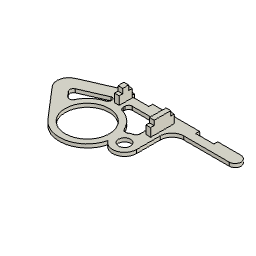
Prototype Body improved v2 (Autodesk Fusion 360 archive; units mm, degrees)
design "bottom_chassis"
Autodesk Fusion 360 part; units mm, degrees
(part 1 of 6)
sketch "Sketch1" plane through (0, 0, 0) normal (0, 0, 1) x (1, 0, 0)
  circle A0 centre (0, 0) radius 18.6
  line L0 (-40.1145, 10.4906) -> (-17.9049, -15.3744)
  line L1 (5, 25.3685) -> (5, 26.9321)
  line L2 (-5, 26.019) -> (-5, 25.3685)
  line L3 (-5, 40) -> (-36.5447, 26.1628)
  line L4 (-28.8171, 18.6328) -> (-7.8034, 27.8505)
  line L5 (-29.888, 13.9311) -> (-26.2116, 9.6495)
  arc A1 (-36.5447, 26.1628) -> (-40.1145, 10.4906) centre (-32.5276, 17.0051) ccw
  line L6 (15.2, 40) -> (15.2, 36.8)
  line L7 (15.2, 36.8) -> (0, 36.8)
  line L8 (0, 36.8) -> (0, 40)
  line L9 (15.2, 40) -> (55, 40)
  line L10 (70.2, 40) -> (70.2, 36.8)
  line L11 (70.2, 36.8) -> (55, 36.8)
  line L12 (55, 36.8) -> (55, 40)
  line L13 (-5, 40) -> (0, 40)
  line L14 (41.6, 0) -> (41.6, 20)
  arc A2 (90, 30) -> (90, 40) centre (90, 35) ccw
  line L15 (90, 30) -> (51.6, 30)
  line L16 (8, 29.9321) -> (28.6, 29.9321)
  line L17 (31.6, 26.9321) -> (31.6, 12.775)
  arc A3 (-17.9049, -15.3744) -> (22.9714, -5.4105) centre (0, 0) ccw
  arc A4 (21.5214, 9.6845) -> (7.0977, 22.5074) centre (0, 0) ccw
  arc A5 (-7.0977, 22.5074) -> (-21.236, 10.2952) centre (0, 0) ccw
  arc A6 (22.9714, -5.4105) -> (41.6, 0) centre (31.5, 0) ccw
  arc A7 (29.2641, 9.8494) -> (25.9158, 8.4159) centre (31.5, 0) ccw
  arc A8 (-28.8171, 18.6328) -> (-29.888, 13.9311) centre (-27.612, 15.8855) ccw
  arc A9 (-26.2116, 9.6495) -> (-21.236, 10.2952) centre (-23.9355, 11.6039) ccw
  arc A10 (-7.0977, 22.5074) -> (-5, 25.3685) centre (-8, 25.3685) ccw
  arc A11 (-5, 26.019) -> (-7.8034, 27.8505) centre (-7, 26.019) ccw
  arc A12 (8, 29.9321) -> (5, 26.9321) centre (8, 26.9321) ccw
  arc A13 (5, 25.3685) -> (7.0977, 22.5074) centre (8, 25.3685) ccw
  arc A14 (21.5214, 9.6845) -> (25.9158, 8.4159) centre (24.2571, 10.9156) ccw
  arc A15 (29.2641, 9.8494) -> (31.6, 12.775) centre (28.6, 12.775) ccw
  arc A16 (31.6, 26.9321) -> (28.6, 29.9321) centre (28.6, 26.9321) ccw
  arc A17 (51.6, 30) -> (41.6, 20) centre (51.6, 20) ccw
  line L18 (0, 40) -> (-5, 40)
  line L19 (90, 40) -> (70.2, 40)
  line L20 (55, 40) -> (15.2, 40)
  line L21 (-2, 36) -> (2, 36)
  line L22 (2, 36) -> (2, 25)
  line L23 (2, 25) -> (-2, 25)
  line L24 (-2, 25) -> (-2, 36)
  line L25 (-2, 33) -> (2, 33)
  line L26 (2, 33) -> (2, 28)
  line L27 (2, 28) -> (-2, 28)
  line L28 (-2, 28) -> (-2, 33)
  line L29 (34.6, 35) -> (38.6, 35)
  line L30 (38.6, 35) -> (38.6, 15)
  line L31 (38.6, 15) -> (34.6, 15)
  line L32 (34.6, 15) -> (34.6, 35)
  line L33 (34.6, 32) -> (38.6, 32)
  line L34 (34.6, 18) -> (38.6, 18)
  circle A18 centre (31.5, 0) radius 5.1
  dimension "d4" = 37.2
  dimension "d6" = 47.2
  dimension "d7" = 20.2
  dimension "d8" = 20
  dimension "d11" = 31.5
  dimension "d12" = 15.2
  dimension "d13" = 3.2
  dimension "d14" = 55
  dimension "d15" = 15.2
  dimension "d16" = 3.2
  dimension "d19" = 3
  dimension "d20" = 2
  dimension "d21" = 3
  dimension "d22" = 10
  dimension "d26" = 4
  dimension "d27" = 20
  dimension "d35" = 10.2
  constraint coincident A0.centre A3.centre
  constraint coincident L0.end A4
  constraint tangent L0 A4
  constraint tangent L0 A1
  constraint parallel L0 L5
  constraint tangent L3 A1
  constraint vertical L6
  constraint horizontal L7
  constraint vertical L8
  constraint perpendicular L6 L9
  constraint vertical L10
  constraint horizontal L11
  constraint vertical L12
  constraint tangent L14 A6
  constraint perpendicular L9 L14
  constraint tangent A2 L19
  constraint tangent A2 L15
  constraint perpendicular L14 L15
  constraint concentric A3 A4
  constraint concentric A4 A5
  constraint concentric A6 A7
  constraint tangent L4 A8
  constraint tangent L5 A8
  constraint tangent L5 A9
  constraint tangent A5 A9
  constraint equal A8 A9
  constraint tangent L2 A10
  constraint tangent A5 A10
  constraint equal A8 A10
  constraint tangent L4 A11
  constraint tangent L2 A11
  constraint tangent L16 A12
  constraint tangent L1 A12
  constraint tangent L1 A13
  constraint tangent A4 A13
  constraint equal A12 A13
  constraint tangent A4 A14
  constraint tangent A7 A14
  constraint equal A12 A14
  constraint tangent L17 A15
  constraint tangent A7 A15
  constraint equal A12 A15
  constraint tangent L16 A16
  constraint tangent L17 A16
  constraint equal A12 A16
  constraint tangent L15 A17
  constraint tangent L14 A17
  constraint collinear L18 L19
  constraint collinear L19 L20
  constraint horizontal L21
  constraint vertical L22
  constraint horizontal L23
  constraint vertical L24
  constraint horizontal L25
  constraint vertical L26
  constraint horizontal L27
  constraint vertical L28
  constraint coincident L22 L26.end
  constraint coincident L24 L25.start
  constraint horizontal L29
  constraint vertical L30
  constraint horizontal L31
  constraint vertical L32
  constraint perpendicular L32 L33
  constraint perpendicular L32 L34
  constraint coincident L30 L34.end
  constraint coincident L32 L34.start
  constraint coincident L32 L33.start
  constraint coincident L30 L33.end
  constraint concentric A6 A18
  measures "d4" diameter of A0
  measures "d6" diameter of A4
  measures "d7" diameter of A6
  measures "d8" diameter of A1
  measures "d11" distance of A0.centre A6.centre
  measures "d12" distance of L8.end L6.start
  measures "d13" distance of L8.end L7.end
  measures "d14" distance of L8.end L9.end
  measures "d15" distance of L9.end L10.start
  measures "d16" distance of L9.end L11.end
  measures "d19" radius of A8
  measures "d20" radius of A11
  measures "d21" radius of A12
  measures "d22" radius of A17
  measures "d26" distance of L29.start L29.end
  measures "d27" distance of L29.start L31.end
  measures "d35" diameter of A18
extrude "Extrude1" add sketch "Sketch1" against normal blind 4 contours L0 L3 A1 L6 L7 L8 L9 L10 L11 L12 L13 L14 A2 L15 A3 A6 A17 L18 L19 L20 | L21 L22 L24 L25 | L22 L24 L25 L26 L27 L28 | L22 L23 L24 L27 | L29 L30 L32 L33 | L30 L32 L33 L34 | L30 L31 L32 L34 | A18
extrude "Extrude2" add sketch "Sketch1" along normal blind 7 contours L21 L22 L24 L25 | L22 L23 L24 L27 | L29 L30 L32 L33 | L30 L31 L32 L34
extrude "Extrude3" add sketch "Sketch1" along normal blind 11 contours L22 L24 L25 L26 L27 L28 | L30 L32 L33 L34
extrude "Extrude4" cut sketch "Sketch1" against normal blind 10 contours A18
extrude "Extrude5" cut 1 faces at (33.2151, 36.6035, -4) along direction (0, 0, 1) blind 1
equation "d6 = 37.200 mm + 5 mm + 5 mm"
equation "d7 = 10.200 mm + 10 mm"
equation "d33 = 7 mm + 4 mm"

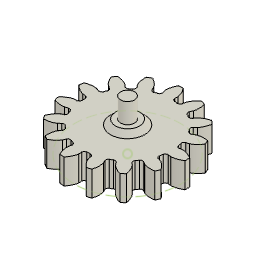
design "motor shaft"
description: Spur Gear; Module: 1.4; Num Teeth: 15; Pressure Angle: 20.0; Backlash: 0.00 mm
Autodesk Fusion 360 part; units mm, degrees
sketch "Sketch1" plane through (0, 0, 0) normal (0, 0, 1) x (1, 0, 0) in component "Spur Gear (15 teeth)"
  circle A0 centre (0, 0) radius 8.7692
  circle A1 centre (0, 0) radius 1.5
extrude "Extrude1" add sketch "Sketch1" along normal blind 5 in component "Spur Gear (15 teeth)"
sketch "Sketch2" plane through (0, 0, 0) normal (0, 0, 1) x (1, 0, 0) in component "Spur Gear (15 teeth)"
  spline S0 degree 5 poles (9.7963, -1.1775) (9.8022, -1.1782) (9.8141, -1.1794) (9.8319, -1.1808) (9.8558, -1.1816) (9.8857, -1.1813) (9.9157, -1.18) (9.9458, -1.1781) (9.9758, -1.1758) (10.0059, -1.1733) (10.0361, -1.1706) (10.0662, -1.1676) (10.0964, -1.1641) (10.1266, -1.1602) (10.1568, -1.1558) (10.187, -1.151) (10.2172, -1.1457) (10.2475, -1.1402) (10.2777, -1.1343) (10.308, -1.1282) (10.3382, -1.1219) (10.3685, -1.1152) (10.3988, -1.1082) (10.429, -1.101) (10.4593, -1.0934) (10.4895, -1.0856) (10.5198, -1.0775) (10.55, -1.0691) (10.5803, -1.0604) (10.6105, -1.0515) (10.6407, -1.0424) (10.671, -1.033) (10.7012, -1.0233) (10.7314, -1.0135) (10.7615, -1.0033) (10.7917, -0.993) (10.8219, -0.9823) (10.852, -0.9715) (10.8821, -0.9604) (10.9122, -0.9491) (10.9423, -0.9376) (10.9724, -0.9258) (11.0024, -0.9139) (11.0325, -0.9017) (11.0625, -0.8893) (11.0925, -0.8766) (11.1224, -0.8638) (11.1524, -0.8508) (11.1823, -0.8375) (11.2122, -0.824) (11.2421, -0.8103) (11.2719, -0.7964) (11.3017, -0.7823) (11.3315, -0.7681) (11.3612, -0.7536) (11.391, -0.7389) (11.4207, -0.724) (11.4503, -0.7089) (11.48, -0.6936) (11.5096, -0.6781) (11.5391, -0.6624) (11.5687, -0.6465) (11.5982, -0.6304) (11.6276, -0.6142) (11.6571, -0.5977) (11.6865, -0.5811) (11.7158, -0.5643) (11.7451, -0.5473) (11.7744, -0.5301) (11.8037, -0.5127) (11.8329, -0.4951) (11.8562, -0.4809) (11.8737, -0.4702) (11.8853, -0.463) (11.8911, -0.4594) knots 0 0 0 0 0 0 0.01428571 0.02857143 0.04285714 0.05714286 0.07142857 0.08571429 0.1 0.11428571 0.12857143 0.14285714 0.15714286 0.17142857 0.18571429 0.2 0.21428571 0.22857143 0.24285714 0.25714286 0.27142857 0.28571429 0.3 0.31428571 0.32857143 0.34285714 0.35714286 0.37142857 0.38571429 0.4 0.41428571 0.42857143 0.44285714 0.45714286 0.47142857 0.48571429 0.5 0.51428571 0.52857143 0.54285714 0.55714286 0.57142857 0.58571429 0.6 0.61428571 0.62857143 0.64285714 0.65714286 0.67142857 0.68571429 0.7 0.71428571 0.72857143 0.74285714 0.75714286 0.77142857 0.78571429 0.8 0.81428571 0.82857143 0.84285714 0.85714286 0.87142857 0.88571429 0.9 0.91428571 0.92857143 0.94285714 0.95714286 0.97142857 0.98571429 1 1 1 1 1 1
  spline S1 degree 5 poles (9.7963, 1.1775) (9.8022, 1.1782) (9.8141, 1.1794) (9.8319, 1.1808) (9.8558, 1.1816) (9.8857, 1.1813) (9.9157, 1.18) (9.9458, 1.1781) (9.9758, 1.1758) (10.0059, 1.1733) (10.0361, 1.1706) (10.0662, 1.1676) (10.0964, 1.1641) (10.1266, 1.1602) (10.1568, 1.1558) (10.187, 1.151) (10.2172, 1.1457) (10.2475, 1.1402) (10.2777, 1.1343) (10.308, 1.1282) (10.3382, 1.1219) (10.3685, 1.1152) (10.3988, 1.1082) (10.429, 1.101) (10.4593, 1.0934) (10.4895, 1.0856) (10.5198, 1.0775) (10.55, 1.0691) (10.5803, 1.0604) (10.6105, 1.0515) (10.6407, 1.0424) (10.671, 1.033) (10.7012, 1.0233) (10.7314, 1.0135) (10.7615, 1.0033) (10.7917, 0.993) (10.8219, 0.9823) (10.852, 0.9715) (10.8821, 0.9604) (10.9122, 0.9491) (10.9423, 0.9376) (10.9724, 0.9258) (11.0024, 0.9139) (11.0325, 0.9017) (11.0625, 0.8893) (11.0925, 0.8766) (11.1224, 0.8638) (11.1524, 0.8508) (11.1823, 0.8375) (11.2122, 0.824) (11.2421, 0.8103) (11.2719, 0.7964) (11.3017, 0.7823) (11.3315, 0.7681) (11.3612, 0.7536) (11.391, 0.7389) (11.4207, 0.724) (11.4503, 0.7089) (11.48, 0.6936) (11.5096, 0.6781) (11.5391, 0.6624) (11.5687, 0.6465) (11.5982, 0.6304) (11.6276, 0.6142) (11.6571, 0.5977) (11.6865, 0.5811) (11.7158, 0.5643) (11.7451, 0.5473) (11.7744, 0.5301) (11.8037, 0.5127) (11.8329, 0.4951) (11.8562, 0.4809) (11.8737, 0.4702) (11.8853, 0.463) (11.8911, 0.4594) knots 0 0 0 0 0 0 0.01428571 0.02857143 0.04285714 0.05714286 0.07142857 0.08571429 0.1 0.11428571 0.12857143 0.14285714 0.15714286 0.17142857 0.18571429 0.2 0.21428571 0.22857143 0.24285714 0.25714286 0.27142857 0.28571429 0.3 0.31428571 0.32857143 0.34285714 0.35714286 0.37142857 0.38571429 0.4 0.41428571 0.42857143 0.44285714 0.45714286 0.47142857 0.48571429 0.5 0.51428571 0.52857143 0.54285714 0.55714286 0.57142857 0.58571429 0.6 0.61428571 0.62857143 0.64285714 0.65714286 0.67142857 0.68571429 0.7 0.71428571 0.72857143 0.74285714 0.75714286 0.77142857 0.78571429 0.8 0.81428571 0.82857143 0.84285714 0.85714286 0.87142857 0.88571429 0.9 0.91428571 0.92857143 0.94285714 0.95714286 0.97142857 0.98571429 1 1 1 1 1 1
  arc A0 (11.8911, -0.4594) -> (11.8911, 0.4594) centre (0, 0) ccw
  line L0 (8.6966, -1.0465) -> (9.7963, -1.1775)
  line L1 (8.6966, 1.0465) -> (9.7963, 1.1775)
  line L2 (8.6966, -1.0465) -> (8.6966, 1.0465)
  point P0 (9.9424, -1.1782)
  point P1 (10.0902, -1.1647)
  point P2 (10.239, -1.1417)
  point P3 (10.3885, -1.1106)
  point P4 (10.5385, -1.0722)
  point P5 (10.6889, -1.0272)
  point P6 (10.8395, -0.976)
  point P7 (10.9903, -0.9187)
  point P8 (11.141, -0.8557)
  point P9 (11.2917, -0.7871)
  point P10 (11.4421, -0.713)
  point P11 (11.5922, -0.6336)
  point P12 (11.7419, -0.5491)
  point P13 (9.9424, 1.1782)
  point P14 (10.0902, 1.1647)
  point P15 (10.239, 1.1417)
  point P16 (10.3885, 1.1106)
  point P17 (10.5385, 1.0722)
  point P18 (10.6889, 1.0272)
  point P19 (10.8395, 0.976)
  point P20 (10.9903, 0.9187)
  point P21 (11.141, 0.8557)
  point P22 (11.2917, 0.7871)
  point P23 (11.4421, 0.713)
  point P24 (11.5922, 0.6336)
  point P25 (11.7419, 0.5491)
extrude "Extrude2" add sketch "Sketch2" along normal blind 5 in component "Spur Gear (15 teeth)"
fillet "Fillet1" radius 0.5 2 edges at (8.7064, -1.0477, 2.5) (8.7064, 1.0477, 2.5) in component "Spur Gear (15 teeth)"
pattern_circular "C-Pattern1" count 15 over 360 about axis through (0, 0, 0) along (0, 0, 1) of "Extrude2", "Fillet1" in component "Spur Gear (15 teeth)"
sketch "Sketch3" plane through (0, 0, 0) normal (0, 0, 1) x (1, 0, 0) in component "Spur Gear (15 teeth)"
  circle A0 centre (0, 0) radius 10.5 construction
sketch "Sketch1 (2)" plane through (0, 0, 5) normal (0, 0, 1) x (-1, 0, 0)
  arc A0 (-8.5069, 2.1289) -> (-8.6373, 1.5152) centre (0, 0) ccw
  arc A1 (-9.1889, 1.1051) -> (-8.6373, 1.5152) centre (-9.1298, 1.6016) ccw
  line L0 (-9.1889, 1.1051) -> (-9.7963, 1.1775)
  spline S0 degree 5 poles (-9.7963, 1.1775) (-9.8022, 1.1782) (-9.8141, 1.1794) (-9.8319, 1.1808) (-9.8558, 1.1816) (-9.8857, 1.1813) (-9.9157, 1.18) (-9.9458, 1.1781) (-9.9758, 1.1758) (-10.0059, 1.1733) (-10.0361, 1.1706) (-10.0662, 1.1676) (-10.0964, 1.1641) (-10.1266, 1.1602) (-10.1568, 1.1558) (-10.187, 1.151) (-10.2172, 1.1457) (-10.2475, 1.1402) (-10.2777, 1.1343) (-10.308, 1.1282) (-10.3382, 1.1219) (-10.3685, 1.1152) (-10.3988, 1.1082) (-10.429, 1.101) (-10.4593, 1.0934) (-10.4895, 1.0856) (-10.5198, 1.0775) (-10.55, 1.0691) (-10.5803, 1.0604) (-10.6105, 1.0515) (-10.6407, 1.0424) (-10.671, 1.033) (-10.7012, 1.0233) (-10.7314, 1.0135) (-10.7615, 1.0033) (-10.7917, 0.993) (-10.8219, 0.9823) (-10.852, 0.9715) (-10.8821, 0.9604) (-10.9122, 0.9491) (-10.9423, 0.9376) (-10.9724, 0.9258) (-11.0024, 0.9139) (-11.0325, 0.9017) (-11.0625, 0.8893) (-11.0925, 0.8766) (-11.1224, 0.8638) (-11.1524, 0.8508) (-11.1823, 0.8375) (-11.2122, 0.824) (-11.2421, 0.8103) (-11.2719, 0.7964) (-11.3017, 0.7823) (-11.3315, 0.7681) (-11.3612, 0.7536) (-11.391, 0.7389) (-11.4207, 0.724) (-11.4503, 0.7089) (-11.48, 0.6936) (-11.5096, 0.6781) (-11.5391, 0.6624) (-11.5687, 0.6465) (-11.5982, 0.6304) (-11.6276, 0.6142) (-11.6571, 0.5977) (-11.6865, 0.5811) (-11.7158, 0.5643) (-11.7451, 0.5473) (-11.7744, 0.5301) (-11.8037, 0.5127) (-11.8329, 0.4951) (-11.8562, 0.4809) (-11.8737, 0.4702) (-11.8853, 0.463) (-11.8911, 0.4594) knots 0 0 0 0 0 0 0.01428571 0.02857143 0.04285714 0.05714286 0.07142857 0.08571429 0.1 0.11428571 0.12857143 0.14285714 0.15714286 0.17142857 0.18571429 0.2 0.21428571 0.22857143 0.24285714 0.25714286 0.27142857 0.28571429 0.3 0.31428571 0.32857143 0.34285714 0.35714286 0.37142857 0.38571429 0.4 0.41428571 0.42857143 0.44285714 0.45714286 0.47142857 0.48571429 0.5 0.51428571 0.52857143 0.54285714 0.55714286 0.57142857 0.58571429 0.6 0.61428571 0.62857143 0.64285714 0.65714286 0.67142857 0.68571429 0.7 0.71428571 0.72857143 0.74285714 0.75714286 0.77142857 0.78571429 0.8 0.81428571 0.82857143 0.84285714 0.85714286 0.87142857 0.88571429 0.9 0.91428571 0.92857143 0.94285714 0.95714286 0.97142857 0.98571429 1 1 1 1 1 1
  arc A2 (-11.8911, 0.4594) -> (-11.8911, -0.4594) centre (0, 0) ccw
  spline S1 degree 5 poles (-11.8911, -0.4594) (-11.8853, -0.463) (-11.8737, -0.4702) (-11.8562, -0.4809) (-11.8329, -0.4951) (-11.8037, -0.5127) (-11.7744, -0.5301) (-11.7451, -0.5473) (-11.7158, -0.5643) (-11.6865, -0.5811) (-11.6571, -0.5977) (-11.6276, -0.6142) (-11.5982, -0.6304) (-11.5687, -0.6465) (-11.5391, -0.6624) (-11.5096, -0.6781) (-11.48, -0.6936) (-11.4503, -0.7089) (-11.4207, -0.724) (-11.391, -0.7389) (-11.3612, -0.7536) (-11.3315, -0.7681) (-11.3017, -0.7823) (-11.2719, -0.7964) (-11.2421, -0.8103) (-11.2122, -0.824) (-11.1823, -0.8375) (-11.1524, -0.8508) (-11.1224, -0.8638) (-11.0925, -0.8766) (-11.0625, -0.8893) (-11.0325, -0.9017) (-11.0024, -0.9139) (-10.9724, -0.9258) (-10.9423, -0.9376) (-10.9122, -0.9491) (-10.8821, -0.9604) (-10.852, -0.9715) (-10.8219, -0.9823) (-10.7917, -0.993) (-10.7615, -1.0033) (-10.7314, -1.0135) (-10.7012, -1.0233) (-10.671, -1.033) (-10.6407, -1.0424) (-10.6105, -1.0515) (-10.5803, -1.0604) (-10.55, -1.0691) (-10.5198, -1.0775) (-10.4895, -1.0856) (-10.4593, -1.0934) (-10.429, -1.101) (-10.3988, -1.1082) (-10.3685, -1.1152) (-10.3382, -1.1219) (-10.308, -1.1282) (-10.2777, -1.1343) (-10.2475, -1.1402) (-10.2172, -1.1457) (-10.187, -1.151) (-10.1568, -1.1558) (-10.1266, -1.1602) (-10.0964, -1.1641) (-10.0662, -1.1676) (-10.0361, -1.1706) (-10.0059, -1.1733) (-9.9758, -1.1758) (-9.9458, -1.1781) (-9.9157, -1.18) (-9.8857, -1.1813) (-9.8558, -1.1816) (-9.8319, -1.1808) (-9.8141, -1.1794) (-9.8022, -1.1782) (-9.7963, -1.1775) knots -1 -1 -1 -1 -1 -1 -0.98571429 -0.97142857 -0.95714286 -0.94285714 -0.92857143 -0.91428571 -0.9 -0.88571429 -0.87142857 -0.85714286 -0.84285714 -0.82857143 -0.81428571 -0.8 -0.78571429 -0.77142857 -0.75714286 -0.74285714 -0.72857143 -0.71428571 -0.7 -0.68571429 -0.67142857 -0.65714286 -0.64285714 -0.62857143 -0.61428571 -0.6 -0.58571429 -0.57142857 -0.55714286 -0.54285714 -0.52857143 -0.51428571 -0.5 -0.48571429 -0.47142857 -0.45714286 -0.44285714 -0.42857143 -0.41428571 -0.4 -0.38571429 -0.37142857 -0.35714286 -0.34285714 -0.32857143 -0.31428571 -0.3 -0.28571429 -0.27142857 -0.25714286 -0.24285714 -0.22857143 -0.21428571 -0.2 -0.18571429 -0.17142857 -0.15714286 -0.14285714 -0.12857143 -0.11428571 -0.1 -0.08571429 -0.07142857 -0.05714286 -0.04285714 -0.02857143 -0.01428571 0 0 0 0 0 0
  line L1 (-9.7963, -1.1775) -> (-9.1889, -1.1051)
  arc A3 (-8.6373, -1.5152) -> (-9.1889, -1.1051) centre (-9.1298, -1.6016) ccw
  arc A4 (-8.6373, -1.5152) -> (-8.5069, -2.1289) centre (0, 0) ccw
  arc A5 (-8.844, -2.7279) -> (-8.5069, -2.1289) centre (-8.9919, -2.2502) ccw
  line L2 (-8.844, -2.7279) -> (-9.4283, -2.9088)
  spline S2 degree 5 poles (-9.4283, -2.9088) (-9.434, -2.9106) (-9.4453, -2.9143) (-9.4622, -2.9203) (-9.4843, -2.9293) (-9.5115, -2.9417) (-9.5384, -2.9551) (-9.5651, -2.9691) (-9.5916, -2.9834) (-9.6181, -2.9979) (-9.6445, -3.0126) (-9.6708, -3.0277) (-9.697, -3.0431) (-9.723, -3.059) (-9.7488, -3.0753) (-9.7744, -3.092) (-9.7999, -3.1091) (-9.8253, -3.1264) (-9.8505, -3.1441) (-9.8757, -3.162) (-9.9008, -3.1801) (-9.9257, -3.1985) (-9.9505, -3.2171) (-9.9752, -3.2361) (-9.9998, -3.2553) (-10.0242, -3.2748) (-10.0485, -3.2945) (-10.0728, -3.3145) (-10.0969, -3.3346) (-10.1209, -3.3551) (-10.1448, -3.3757) (-10.1686, -3.3966) (-10.1922, -3.4177) (-10.2158, -3.439) (-10.2392, -3.4605) (-10.2626, -3.4823) (-10.2858, -3.5042) (-10.3089, -3.5264) (-10.332, -3.5488) (-10.3549, -3.5713) (-10.3777, -3.5941) (-10.4004, -3.6171) (-10.4229, -3.6402) (-10.4454, -3.6636) (-10.4678, -3.6871) (-10.49, -3.7109) (-10.5122, -3.7348) (-10.5342, -3.7589) (-10.5562, -3.7832) (-10.578, -3.8076) (-10.5997, -3.8323) (-10.6213, -3.8571) (-10.6428, -3.8821) (-10.6642, -3.9073) (-10.6855, -3.9326) (-10.7067, -3.9581) (-10.7278, -3.9838) (-10.7487, -4.0097) (-10.7696, -4.0357) (-10.7903, -4.0619) (-10.8109, -4.0883) (-10.8315, -4.1148) (-10.8519, -4.1415) (-10.8722, -4.1683) (-10.8924, -4.1953) (-10.9125, -4.2225) (-10.9324, -4.2498) (-10.9523, -4.2772) (-10.9721, -4.3049) (-10.9917, -4.3326) (-11.0112, -4.3606) (-11.0268, -4.383) (-11.0384, -4.3999) (-11.0461, -4.4113) (-11.0499, -4.4169) knots 0 0 0 0 0 0 0.01428571 0.02857143 0.04285714 0.05714286 0.07142857 0.08571429 0.1 0.11428571 0.12857143 0.14285714 0.15714286 0.17142857 0.18571429 0.2 0.21428571 0.22857143 0.24285714 0.25714286 0.27142857 0.28571429 0.3 0.31428571 0.32857143 0.34285714 0.35714286 0.37142857 0.38571429 0.4 0.41428571 0.42857143 0.44285714 0.45714286 0.47142857 0.48571429 0.5 0.51428571 0.52857143 0.54285714 0.55714286 0.57142857 0.58571429 0.6 0.61428571 0.62857143 0.64285714 0.65714286 0.67142857 0.68571429 0.7 0.71428571 0.72857143 0.74285714 0.75714286 0.77142857 0.78571429 0.8 0.81428571 0.82857143 0.84285714 0.85714286 0.87142857 0.88571429 0.9 0.91428571 0.92857143 0.94285714 0.95714286 0.97142857 0.98571429 1 1 1 1 1 1
  arc A6 (-11.0499, -4.4169) -> (-10.6762, -5.2562) centre (0, 0) ccw
  spline S3 degree 5 poles (-10.6762, -5.2562) (-10.6695, -5.2571) (-10.6559, -5.259) (-10.6356, -5.2617) (-10.6085, -5.2652) (-10.5747, -5.2693) (-10.5409, -5.2733) (-10.5071, -5.2771) (-10.4734, -5.2807) (-10.4398, -5.2842) (-10.4061, -5.2874) (-10.3726, -5.2905) (-10.339, -5.2933) (-10.3055, -5.296) (-10.2721, -5.2985) (-10.2387, -5.3008) (-10.2054, -5.3029) (-10.1721, -5.3048) (-10.1388, -5.3066) (-10.1057, -5.3081) (-10.0725, -5.3094) (-10.0394, -5.3106) (-10.0064, -5.3115) (-9.9734, -5.3123) (-9.9405, -5.3128) (-9.9077, -5.3132) (-9.8749, -5.3133) (-9.8422, -5.3133) (-9.8095, -5.313) (-9.7769, -5.3126) (-9.7444, -5.3119) (-9.7119, -5.311) (-9.6795, -5.31) (-9.6472, -5.3087) (-9.615, -5.3072) (-9.5828, -5.3055) (-9.5507, -5.3035) (-9.5187, -5.3014) (-9.4867, -5.2991) (-9.4548, -5.2965) (-9.4231, -5.2937) (-9.3914, -5.2907) (-9.3598, -5.2874) (-9.3282, -5.2839) (-9.2968, -5.2802) (-9.2655, -5.2763) (-9.2343, -5.2721) (-9.2031, -5.2677) (-9.1721, -5.2631) (-9.1411, -5.2582) (-9.1103, -5.2531) (-9.0796, -5.2477) (-9.049, -5.242) (-9.0185, -5.236) (-8.9882, -5.2298) (-8.9579, -5.2233) (-8.9278, -5.2166) (-8.8978, -5.2096) (-8.8679, -5.2024) (-8.8382, -5.1949) (-8.8086, -5.187) (-8.7792, -5.1787) (-8.75, -5.17) (-8.7211, -5.1609) (-8.6923, -5.1514) (-8.6637, -5.1417) (-8.6351, -5.1317) (-8.6068, -5.1215) (-8.5785, -5.111) (-8.5506, -5.1) (-8.5231, -5.0882) (-8.5017, -5.0777) (-8.4859, -5.0692) (-8.4755, -5.0633) (-8.4704, -5.0602) knots -1 -1 -1 -1 -1 -1 -0.98571429 -0.97142857 -0.95714286 -0.94285714 -0.92857143 -0.91428571 -0.9 -0.88571429 -0.87142857 -0.85714286 -0.84285714 -0.82857143 -0.81428571 -0.8 -0.78571429 -0.77142857 -0.75714286 -0.74285714 -0.72857143 -0.71428571 -0.7 -0.68571429 -0.67142857 -0.65714286 -0.64285714 -0.62857143 -0.61428571 -0.6 -0.58571429 -0.57142857 -0.55714286 -0.54285714 -0.52857143 -0.51428571 -0.5 -0.48571429 -0.47142857 -0.45714286 -0.44285714 -0.42857143 -0.41428571 -0.4 -0.38571429 -0.37142857 -0.35714286 -0.34285714 -0.32857143 -0.31428571 -0.3 -0.28571429 -0.27142857 -0.25714286 -0.24285714 -0.22857143 -0.21428571 -0.2 -0.18571429 -0.17142857 -0.15714286 -0.14285714 -0.12857143 -0.11428571 -0.1 -0.08571429 -0.07142857 -0.05714286 -0.04285714 -0.02857143 -0.01428571 0 0 0 0 0 0
  line L3 (-8.4704, -5.0602) -> (-7.945, -4.7471)
  arc A7 (-7.2743, -4.8973) -> (-7.945, -4.7471) centre (-7.689, -5.1766) ccw
  arc A8 (-7.2743, -4.8973) -> (-6.9055, -5.4049) centre (0, 0) ccw
  arc A9 (-6.9699, -6.0892) -> (-6.9055, -5.4049) centre (-7.2993, -5.713) ccw
  line L4 (-6.9699, -6.0892) -> (-7.43, -6.4921)
  spline S4 degree 5 poles (-7.43, -6.4921) (-7.4345, -6.4961) (-7.4434, -6.5041) (-7.4563, -6.5165) (-7.4729, -6.5336) (-7.4927, -6.5561) (-7.5118, -6.5793) (-7.5305, -6.6029) (-7.5489, -6.6267) (-7.5672, -6.6508) (-7.5854, -6.675) (-7.6033, -6.6994) (-7.6209, -6.7241) (-7.6382, -6.7492) (-7.6551, -6.7746) (-7.6718, -6.8003) (-7.6881, -6.8262) (-7.7042, -6.8524) (-7.7201, -6.8788) (-7.7358, -6.9054) (-7.7513, -6.9321) (-7.7666, -6.9591) (-7.7817, -6.9862) (-7.7966, -7.0136) (-7.8112, -7.0411) (-7.8256, -7.0688) (-7.8398, -7.0968) (-7.8538, -7.1249) (-7.8676, -7.1531) (-7.8813, -7.1815) (-7.8947, -7.2101) (-7.9079, -7.2389) (-7.921, -7.2678) (-7.9338, -7.2968) (-7.9465, -7.326) (-7.959, -7.3554) (-7.9713, -7.3849) (-7.9834, -7.4146) (-7.9953, -7.4443) (-8.007, -7.4743) (-8.0186, -7.5044) (-8.03, -7.5346) (-8.0412, -7.5649) (-8.0522, -7.5954) (-8.0631, -7.626) (-8.0738, -7.6567) (-8.0843, -7.6876) (-8.0946, -7.7186) (-8.1048, -7.7497) (-8.1148, -7.7809) (-8.1246, -7.8123) (-8.1342, -7.8437) (-8.1437, -7.8753) (-8.153, -7.907) (-8.1622, -7.9388) (-8.1711, -7.9708) (-8.1799, -8.0028) (-8.1886, -8.0349) (-8.197, -8.0672) (-8.2053, -8.0996) (-8.2134, -8.132) (-8.2214, -8.1646) (-8.2292, -8.1973) (-8.2368, -8.2301) (-8.2443, -8.2629) (-8.2516, -8.2959) (-8.2587, -8.329) (-8.2657, -8.3622) (-8.2725, -8.3954) (-8.2792, -8.4288) (-8.2857, -8.4622) (-8.2907, -8.4891) (-8.2944, -8.5093) (-8.2969, -8.5227) (-8.2981, -8.5295) knots 0 0 0 0 0 0 0.01428571 0.02857143 0.04285714 0.05714286 0.07142857 0.08571429 0.1 0.11428571 0.12857143 0.14285714 0.15714286 0.17142857 0.18571429 0.2 0.21428571 0.22857143 0.24285714 0.25714286 0.27142857 0.28571429 0.3 0.31428571 0.32857143 0.34285714 0.35714286 0.37142857 0.38571429 0.4 0.41428571 0.42857143 0.44285714 0.45714286 0.47142857 0.48571429 0.5 0.51428571 0.52857143 0.54285714 0.55714286 0.57142857 0.58571429 0.6 0.61428571 0.62857143 0.64285714 0.65714286 0.67142857 0.68571429 0.7 0.71428571 0.72857143 0.74285714 0.75714286 0.77142857 0.78571429 0.8 0.81428571 0.82857143 0.84285714 0.85714286 0.87142857 0.88571429 0.9 0.91428571 0.92857143 0.94285714 0.95714286 0.97142857 0.98571429 1 1 1 1 1 1
  arc A10 (-8.2981, -8.5295) -> (-7.6153, -9.1442) centre (0, 0) ccw
  spline S5 degree 5 poles (-7.6153, -9.1442) (-7.6088, -9.1423) (-7.5956, -9.1385) (-7.576, -9.1326) (-7.5498, -9.1248) (-7.5172, -9.1149) (-7.4847, -9.1048) (-7.4523, -9.0945) (-7.4201, -9.0841) (-7.3879, -9.0736) (-7.3559, -9.0629) (-7.324, -9.052) (-7.2922, -9.041) (-7.2605, -9.0298) (-7.2289, -9.0185) (-7.1975, -9.007) (-7.1662, -8.9954) (-7.135, -8.9836) (-7.1039, -8.9716) (-7.073, -8.9595) (-7.0422, -8.9473) (-7.0115, -8.9349) (-6.9809, -8.9223) (-6.9505, -8.9096) (-6.9202, -8.8967) (-6.8901, -8.8837) (-6.86, -8.8705) (-6.8302, -8.8571) (-6.8004, -8.8436) (-6.7708, -8.8299) (-6.7414, -8.8161) (-6.7121, -8.8021) (-6.6829, -8.7879) (-6.6539, -8.7736) (-6.6251, -8.7591) (-6.5964, -8.7445) (-6.5678, -8.7296) (-6.5394, -8.7147) (-6.5112, -8.6995) (-6.4832, -8.6842) (-6.4553, -8.6687) (-6.4275, -8.6531) (-6.4, -8.6373) (-6.3726, -8.6213) (-6.3454, -8.6051) (-6.3184, -8.5888) (-6.2915, -8.5722) (-6.2649, -8.5555) (-6.2384, -8.5387) (-6.2121, -8.5216) (-6.186, -8.5044) (-6.1602, -8.487) (-6.1345, -8.4693) (-6.1091, -8.4515) (-6.0839, -8.4335) (-6.059, -8.4153) (-6.0342, -8.3969) (-6.0096, -8.3783) (-5.9852, -8.3595) (-5.9611, -8.3406) (-5.9373, -8.3213) (-5.9138, -8.3018) (-5.8907, -8.282) (-5.868, -8.2619) (-5.8455, -8.2415) (-5.8233, -8.221) (-5.8014, -8.2003) (-5.7796, -8.1794) (-5.758, -8.1584) (-5.737, -8.137) (-5.7167, -8.1149) (-5.7014, -8.0967) (-5.6904, -8.0825) (-5.6834, -8.0728) (-5.6799, -8.0679) knots -1 -1 -1 -1 -1 -1 -0.98571429 -0.97142857 -0.95714286 -0.94285714 -0.92857143 -0.91428571 -0.9 -0.88571429 -0.87142857 -0.85714286 -0.84285714 -0.82857143 -0.81428571 -0.8 -0.78571429 -0.77142857 -0.75714286 -0.74285714 -0.72857143 -0.71428571 -0.7 -0.68571429 -0.67142857 -0.65714286 -0.64285714 -0.62857143 -0.61428571 -0.6 -0.58571429 -0.57142857 -0.55714286 -0.54285714 -0.52857143 -0.51428571 -0.5 -0.48571429 -0.47142857 -0.45714286 -0.44285714 -0.42857143 -0.41428571 -0.4 -0.38571429 -0.37142857 -0.35714286 -0.34285714 -0.32857143 -0.31428571 -0.3 -0.28571429 -0.27142857 -0.25714286 -0.24285714 -0.22857143 -0.21428571 -0.2 -0.18571429 -0.17142857 -0.15714286 -0.14285714 -0.12857143 -0.11428571 -0.1 -0.08571429 -0.07142857 -0.05714286 -0.04285714 -0.02857143 -0.01428571 0 0 0 0 0 0
  line L5 (-5.6799, -8.0679) -> (-5.3273, -7.5682)
  arc A11 (-4.6534, -7.4327) -> (-5.3273, -7.5682) centre (-4.9188, -7.8565) ccw
  arc A12 (-4.6534, -7.4327) -> (-4.1102, -7.7463) centre (0, 0) ccw
  arc A13 (-3.8906, -8.3977) -> (-4.1102, -7.7463) centre (-4.3445, -8.188) ccw
  line L6 (-3.8906, -8.3977) -> (-4.1471, -8.9529)
  spline S6 degree 5 poles (-4.1471, -8.9529) (-4.1496, -8.9584) (-4.1544, -8.9693) (-4.1612, -8.9858) (-4.1694, -9.0083) (-4.1783, -9.0369) (-4.1863, -9.0658) (-4.1938, -9.0949) (-4.201, -9.1243) (-4.2079, -9.1536) (-4.2146, -9.1831) (-4.221, -9.2127) (-4.2271, -9.2425) (-4.2327, -9.2724) (-4.2378, -9.3025) (-4.2426, -9.3328) (-4.2469, -9.3631) (-4.251, -9.3936) (-4.2548, -9.4242) (-4.2583, -9.4548) (-4.2616, -9.4856) (-4.2647, -9.5164) (-4.2674, -9.5473) (-4.2698, -9.5784) (-4.272, -9.6095) (-4.2739, -9.6407) (-4.2755, -9.672) (-4.2769, -9.7033) (-4.278, -9.7348) (-4.2789, -9.7663) (-4.2795, -9.7978) (-4.2799, -9.8295) (-4.2801, -9.8612) (-4.28, -9.8929) (-4.2797, -9.9248) (-4.2792, -9.9567) (-4.2784, -9.9886) (-4.2774, -10.0207) (-4.2762, -10.0527) (-4.2747, -10.0849) (-4.2731, -10.117) (-4.2712, -10.1493) (-4.2691, -10.1815) (-4.2668, -10.2139) (-4.2642, -10.2462) (-4.2615, -10.2787) (-4.2586, -10.3111) (-4.2554, -10.3436) (-4.252, -10.3762) (-4.2484, -10.4088) (-4.2447, -10.4414) (-4.2407, -10.4741) (-4.2365, -10.5068) (-4.2321, -10.5395) (-4.2275, -10.5723) (-4.2227, -10.6051) (-4.2177, -10.638) (-4.2125, -10.6709) (-4.2071, -10.7038) (-4.2015, -10.7367) (-4.1958, -10.7697) (-4.1898, -10.8027) (-4.1836, -10.8357) (-4.1773, -10.8688) (-4.1707, -10.9018) (-4.164, -10.9349) (-4.157, -10.968) (-4.1499, -11.0012) (-4.1426, -11.0343) (-4.1351, -11.0675) (-4.1274, -11.1007) (-4.1211, -11.1273) (-4.1163, -11.1472) (-4.1131, -11.1605) (-4.1114, -11.1672) knots 0 0 0 0 0 0 0.01428571 0.02857143 0.04285714 0.05714286 0.07142857 0.08571429 0.1 0.11428571 0.12857143 0.14285714 0.15714286 0.17142857 0.18571429 0.2 0.21428571 0.22857143 0.24285714 0.25714286 0.27142857 0.28571429 0.3 0.31428571 0.32857143 0.34285714 0.35714286 0.37142857 0.38571429 0.4 0.41428571 0.42857143 0.44285714 0.45714286 0.47142857 0.48571429 0.5 0.51428571 0.52857143 0.54285714 0.55714286 0.57142857 0.58571429 0.6 0.61428571 0.62857143 0.64285714 0.65714286 0.67142857 0.68571429 0.7 0.71428571 0.72857143 0.74285714 0.75714286 0.77142857 0.78571429 0.8 0.81428571 0.82857143 0.84285714 0.85714286 0.87142857 0.88571429 0.9 0.91428571 0.92857143 0.94285714 0.95714286 0.97142857 0.98571429 1 1 1 1 1 1
  arc A14 (-4.1114, -11.1672) -> (-3.2377, -11.4511) centre (0, 0) ccw
  spline S7 degree 5 poles (-3.2377, -11.4511) (-3.2325, -11.4467) (-3.222, -11.4378) (-3.2064, -11.4245) (-3.1857, -11.4067) (-3.16, -11.3844) (-3.1344, -11.3619) (-3.109, -11.3394) (-3.0837, -11.3168) (-3.0587, -11.2941) (-3.0338, -11.2712) (-3.009, -11.2483) (-2.9844, -11.2253) (-2.96, -11.2022) (-2.9358, -11.1791) (-2.9118, -11.1558) (-2.8879, -11.1324) (-2.8642, -11.109) (-2.8407, -11.0854) (-2.8173, -11.0618) (-2.7941, -11.0381) (-2.7712, -11.0142) (-2.7484, -10.9903) (-2.7257, -10.9663) (-2.7033, -10.9422) (-2.6811, -10.9181) (-2.659, -10.8938) (-2.6372, -10.8694) (-2.6155, -10.845) (-2.594, -10.8205) (-2.5727, -10.7958) (-2.5517, -10.7711) (-2.5308, -10.7463) (-2.5101, -10.7215) (-2.4897, -10.6965) (-2.4694, -10.6714) (-2.4493, -10.6463) (-2.4295, -10.6211) (-2.4099, -10.5958) (-2.3905, -10.5704) (-2.3713, -10.5449) (-2.3523, -10.5193) (-2.3336, -10.4936) (-2.3151, -10.4679) (-2.2968, -10.4421) (-2.2788, -10.4161) (-2.261, -10.3901) (-2.2434, -10.364) (-2.2261, -10.3379) (-2.209, -10.3116) (-2.1922, -10.2853) (-2.1756, -10.2588) (-2.1594, -10.2323) (-2.1434, -10.2056) (-2.1277, -10.1789) (-2.1123, -10.1521) (-2.0972, -10.1252) (-2.0823, -10.0983) (-2.0677, -10.0712) (-2.0533, -10.0441) (-2.0394, -10.0168) (-2.0259, -9.9895) (-2.0128, -9.962) (-2.0002, -9.9343) (-1.988, -9.9066) (-1.9761, -9.8788) (-1.9645, -9.8509) (-1.953, -9.823) (-1.9419, -9.795) (-1.9314, -9.7669) (-1.9218, -9.7386) (-1.9152, -9.7156) (-1.911, -9.6982) (-1.9085, -9.6865) (-1.9074, -9.6807) knots -1 -1 -1 -1 -1 -1 -0.98571429 -0.97142857 -0.95714286 -0.94285714 -0.92857143 -0.91428571 -0.9 -0.88571429 -0.87142857 -0.85714286 -0.84285714 -0.82857143 -0.81428571 -0.8 -0.78571429 -0.77142857 -0.75714286 -0.74285714 -0.72857143 -0.71428571 -0.7 -0.68571429 -0.67142857 -0.65714286 -0.64285714 -0.62857143 -0.61428571 -0.6 -0.58571429 -0.57142857 -0.55714286 -0.54285714 -0.52857143 -0.51428571 -0.5 -0.48571429 -0.47142857 -0.45714286 -0.44285714 -0.42857143 -0.41428571 -0.4 -0.38571429 -0.37142857 -0.35714286 -0.34285714 -0.32857143 -0.31428571 -0.3 -0.28571429 -0.27142857 -0.25714286 -0.24285714 -0.22857143 -0.21428571 -0.2 -0.18571429 -0.17142857 -0.15714286 -0.14285714 -0.12857143 -0.11428571 -0.1 -0.08571429 -0.07142857 -0.05714286 -0.04285714 -0.02857143 -0.01428571 0 0 0 0 0 0
  line L7 (-1.9074, -9.6807) -> (-1.7885, -9.0807)
  arc A15 (-1.228, -8.6828) -> (-1.7885, -9.0807) centre (-1.298, -9.1779) ccw
  arc A16 (-1.228, -8.6828) -> (-0.6041, -8.7484) centre (0, 0) ccw
  arc A17 (-0.1386, -9.2541) -> (-0.6041, -8.7484) centre (-0.6385, -9.2472) ccw
  line L8 (-0.1386, -9.2541) -> (-0.1471, -9.8657)
  spline S8 degree 5 poles (-0.1471, -9.8657) (-0.1471, -9.8717) (-0.1471, -9.8836) (-0.1466, -9.9015) (-0.1449, -9.9253) (-0.1415, -9.9551) (-0.137, -9.9847) (-0.132, -10.0144) (-0.1266, -10.0441) (-0.121, -10.0738) (-0.1151, -10.1035) (-0.109, -10.1331) (-0.1024, -10.1628) (-0.0953, -10.1924) (-0.0878, -10.222) (-0.0798, -10.2515) (-0.0715, -10.281) (-0.0628, -10.3105) (-0.0538, -10.34) (-0.0446, -10.3694) (-0.0351, -10.3989) (-0.0253, -10.4283) (-0.0152, -10.4576) (-0.0048, -10.487) (0.0059, -10.5163) (0.0168, -10.5455) (0.0281, -10.5748) (0.0396, -10.604) (0.0513, -10.6332) (0.0633, -10.6623) (0.0756, -10.6914) (0.0881, -10.7205) (0.1008, -10.7495) (0.1138, -10.7785) (0.1271, -10.8075) (0.1405, -10.8364) (0.1542, -10.8653) (0.1682, -10.8941) (0.1823, -10.9229) (0.1967, -10.9517) (0.2113, -10.9804) (0.2262, -11.0091) (0.2412, -11.0377) (0.2565, -11.0663) (0.2719, -11.0948) (0.2876, -11.1233) (0.3035, -11.1518) (0.3196, -11.1802) (0.336, -11.2086) (0.3525, -11.2369) (0.3692, -11.2652) (0.3862, -11.2934) (0.4033, -11.3216) (0.4206, -11.3497) (0.4381, -11.3778) (0.4559, -11.4058) (0.4738, -11.4338) (0.4919, -11.4617) (0.5102, -11.4896) (0.5287, -11.5174) (0.5474, -11.5452) (0.5663, -11.5729) (0.5853, -11.6005) (0.6046, -11.6281) (0.624, -11.6557) (0.6437, -11.6832) (0.6635, -11.7106) (0.6834, -11.738) (0.7036, -11.7653) (0.724, -11.7926) (0.7445, -11.8198) (0.761, -11.8415) (0.7736, -11.8578) (0.7819, -11.8686) (0.7861, -11.874) knots 0 0 0 0 0 0 0.01428571 0.02857143 0.04285714 0.05714286 0.07142857 0.08571429 0.1 0.11428571 0.12857143 0.14285714 0.15714286 0.17142857 0.18571429 0.2 0.21428571 0.22857143 0.24285714 0.25714286 0.27142857 0.28571429 0.3 0.31428571 0.32857143 0.34285714 0.35714286 0.37142857 0.38571429 0.4 0.41428571 0.42857143 0.44285714 0.45714286 0.47142857 0.48571429 0.5 0.51428571 0.52857143 0.54285714 0.55714286 0.57142857 0.58571429 0.6 0.61428571 0.62857143 0.64285714 0.65714286 0.67142857 0.68571429 0.7 0.71428571 0.72857143 0.74285714 0.75714286 0.77142857 0.78571429 0.8 0.81428571 0.82857143 0.84285714 0.85714286 0.87142857 0.88571429 0.9 0.91428571 0.92857143 0.94285714 0.95714286 0.97142857 0.98571429 1 1 1 1 1 1
  arc A18 (0.7861, -11.874) -> (1.6998, -11.778) centre (0, 0) ccw
  spline S9 degree 5 poles (1.6998, -11.778) (1.7028, -11.7718) (1.7087, -11.7595) (1.7176, -11.741) (1.7293, -11.7163) (1.7437, -11.6854) (1.7579, -11.6545) (1.772, -11.6236) (1.7858, -11.5927) (1.7995, -11.5617) (1.813, -11.5307) (1.8262, -11.4997) (1.8393, -11.4687) (1.8522, -11.4377) (1.8649, -11.4067) (1.8774, -11.3756) (1.8897, -11.3446) (1.9019, -11.3135) (1.9138, -11.2824) (1.9255, -11.2513) (1.937, -11.2202) (1.9483, -11.1891) (1.9594, -11.158) (1.9703, -11.1269) (1.981, -11.0958) (1.9915, -11.0646) (2.0018, -11.0335) (2.0118, -11.0024) (2.0217, -10.9712) (2.0313, -10.9401) (2.0407, -10.9089) (2.05, -10.8778) (2.0589, -10.8466) (2.0677, -10.8155) (2.0762, -10.7844) (2.0846, -10.7532) (2.0927, -10.7221) (2.1005, -10.691) (2.1082, -10.6599) (2.1156, -10.6288) (2.1227, -10.5977) (2.1296, -10.5666) (2.1363, -10.5356) (2.1427, -10.5045) (2.1489, -10.4735) (2.1549, -10.4425) (2.1605, -10.4115) (2.166, -10.3805) (2.1712, -10.3495) (2.1761, -10.3186) (2.1807, -10.2877) (2.1851, -10.2568) (2.1891, -10.226) (2.1929, -10.1951) (2.1963, -10.1643) (2.1995, -10.1336) (2.2024, -10.1029) (2.2051, -10.0722) (2.2074, -10.0415) (2.2095, -10.0109) (2.2111, -9.9803) (2.2124, -9.9498) (2.2131, -9.9194) (2.2134, -9.889) (2.2132, -9.8587) (2.2128, -9.8285) (2.2121, -9.7983) (2.2112, -9.7681) (2.21, -9.7381) (2.2081, -9.7081) (2.2053, -9.6783) (2.202, -9.6547) (2.1988, -9.637) (2.1964, -9.6253) (2.195, -9.6195) knots -1 -1 -1 -1 -1 -1 -0.98571429 -0.97142857 -0.95714286 -0.94285714 -0.92857143 -0.91428571 -0.9 -0.88571429 -0.87142857 -0.85714286 -0.84285714 -0.82857143 -0.81428571 -0.8 -0.78571429 -0.77142857 -0.75714286 -0.74285714 -0.72857143 -0.71428571 -0.7 -0.68571429 -0.67142857 -0.65714286 -0.64285714 -0.62857143 -0.61428571 -0.6 -0.58571429 -0.57142857 -0.55714286 -0.54285714 -0.52857143 -0.51428571 -0.5 -0.48571429 -0.47142857 -0.45714286 -0.44285714 -0.42857143 -0.41428571 -0.4 -0.38571429 -0.37142857 -0.35714286 -0.34285714 -0.32857143 -0.31428571 -0.3 -0.28571429 -0.27142857 -0.25714286 -0.24285714 -0.22857143 -0.21428571 -0.2 -0.18571429 -0.17142857 -0.15714286 -0.14285714 -0.12857143 -0.11428571 -0.1 -0.08571429 -0.07142857 -0.05714286 -0.04285714 -0.02857143 -0.01428571 0 0 0 0 0 0
  line L9 (2.195, -9.6195) -> (2.0596, -9.0231)
  arc A19 (2.4098, -8.4316) -> (2.0596, -9.0231) centre (2.5472, -8.9123) ccw
  arc A20 (2.4098, -8.4316) -> (3.0064, -8.2377) centre (0, 0) ccw
  arc A21 (3.6374, -8.5104) -> (3.0064, -8.2377) centre (3.1778, -8.7074) ccw
  line L10 (3.6374, -8.5104) -> (3.8784, -9.0726)
  spline S10 degree 5 poles (3.8784, -9.0726) (3.8807, -9.0781) (3.8856, -9.089) (3.8934, -9.1051) (3.9046, -9.1262) (3.9199, -9.1519) (3.936, -9.1773) (3.9527, -9.2023) (3.9696, -9.2272) (3.9869, -9.2521) (4.0043, -9.2768) (4.022, -9.3014) (4.04, -9.3258) (4.0585, -9.35) (4.0774, -9.3739) (4.0967, -9.3977) (4.1164, -9.4213) (4.1363, -9.4447) (4.1565, -9.4679) (4.1769, -9.4911) (4.1976, -9.5141) (4.2185, -9.537) (4.2396, -9.5597) (4.261, -9.5823) (4.2827, -9.6047) (4.3046, -9.627) (4.3268, -9.6491) (4.3492, -9.6711) (4.3718, -9.693) (4.3946, -9.7147) (4.4176, -9.7363) (4.4409, -9.7578) (4.4643, -9.7792) (4.488, -9.8004) (4.5119, -9.8214) (4.5359, -9.8424) (4.5602, -9.8632) (4.5847, -9.8839) (4.6093, -9.9044) (4.6342, -9.9248) (4.6592, -9.9451) (4.6844, -9.9653) (4.7098, -9.9853) (4.7354, -10.0052) (4.7611, -10.025) (4.787, -10.0447) (4.8131, -10.0642) (4.8394, -10.0836) (4.8659, -10.1029) (4.8925, -10.122) (4.9193, -10.1411) (4.9462, -10.16) (4.9733, -10.1787) (5.0006, -10.1974) (5.028, -10.2159) (5.0556, -10.2343) (5.0834, -10.2526) (5.1113, -10.2707) (5.1393, -10.2887) (5.1676, -10.3066) (5.1959, -10.3244) (5.2244, -10.342) (5.2531, -10.3595) (5.2819, -10.3769) (5.3109, -10.3942) (5.34, -10.4113) (5.3692, -10.4283) (5.3986, -10.4452) (5.4282, -10.462) (5.4578, -10.4786) (5.4877, -10.4951) (5.5116, -10.5082) (5.5297, -10.518) (5.5417, -10.5245) (5.5477, -10.5277) knots 0 0 0 0 0 0 0.01428571 0.02857143 0.04285714 0.05714286 0.07142857 0.08571429 0.1 0.11428571 0.12857143 0.14285714 0.15714286 0.17142857 0.18571429 0.2 0.21428571 0.22857143 0.24285714 0.25714286 0.27142857 0.28571429 0.3 0.31428571 0.32857143 0.34285714 0.35714286 0.37142857 0.38571429 0.4 0.41428571 0.42857143 0.44285714 0.45714286 0.47142857 0.48571429 0.5 0.51428571 0.52857143 0.54285714 0.55714286 0.57142857 0.58571429 0.6 0.61428571 0.62857143 0.64285714 0.65714286 0.67142857 0.68571429 0.7 0.71428571 0.72857143 0.74285714 0.75714286 0.77142857 0.78571429 0.8 0.81428571 0.82857143 0.84285714 0.85714286 0.87142857 0.88571429 0.9 0.91428571 0.92857143 0.94285714 0.95714286 0.97142857 0.98571429 1 1 1 1 1 1
  arc A22 (5.5477, -10.5277) -> (6.3434, -10.0683) centre (0, 0) ccw
  spline S11 degree 5 poles (6.3434, -10.0683) (6.3436, -10.0615) (6.344, -10.0478) (6.3446, -10.0273) (6.3452, -10) (6.3458, -9.9659) (6.3462, -9.9319) (6.3465, -9.898) (6.3466, -9.8641) (6.3465, -9.8302) (6.3462, -9.7965) (6.3457, -9.7627) (6.3451, -9.7291) (6.3442, -9.6955) (6.3432, -9.662) (6.342, -9.6285) (6.3406, -9.5952) (6.3391, -9.5619) (6.3373, -9.5286) (6.3354, -9.4954) (6.3332, -9.4624) (6.3309, -9.4293) (6.3284, -9.3964) (6.3257, -9.3635) (6.3228, -9.3307) (6.3197, -9.298) (6.3164, -9.2654) (6.313, -9.2329) (6.3093, -9.2004) (6.3054, -9.168) (6.3014, -9.1358) (6.2971, -9.1036) (6.2927, -9.0715) (6.288, -9.0394) (6.2831, -9.0075) (6.2781, -8.9757) (6.2728, -8.944) (6.2673, -8.9124) (6.2617, -8.8808) (6.2558, -8.8494) (6.2497, -8.8181) (6.2434, -8.7869) (6.2368, -8.7558) (6.2301, -8.7248) (6.2231, -8.694) (6.2159, -8.6632) (6.2085, -8.6326) (6.2009, -8.6021) (6.193, -8.5717) (6.1849, -8.5414) (6.1766, -8.5113) (6.168, -8.4813) (6.1591, -8.4515) (6.15, -8.4218) (6.1407, -8.3923) (6.1311, -8.3629) (6.1212, -8.3336) (6.1112, -8.3045) (6.1008, -8.2755) (6.0903, -8.2467) (6.0793, -8.2181) (6.068, -8.1898) (6.0563, -8.1617) (6.0442, -8.1338) (6.0318, -8.1062) (6.0191, -8.0787) (6.0062, -8.0514) (5.9931, -8.0243) (5.9797, -7.9973) (5.9659, -7.9707) (5.9512, -7.9446) (5.9386, -7.9243) (5.9285, -7.9095) (5.9214, -7.8999) (5.9179, -7.8951) knots -1 -1 -1 -1 -1 -1 -0.98571429 -0.97142857 -0.95714286 -0.94285714 -0.92857143 -0.91428571 -0.9 -0.88571429 -0.87142857 -0.85714286 -0.84285714 -0.82857143 -0.81428571 -0.8 -0.78571429 -0.77142857 -0.75714286 -0.74285714 -0.72857143 -0.71428571 -0.7 -0.68571429 -0.67142857 -0.65714286 -0.64285714 -0.62857143 -0.61428571 -0.6 -0.58571429 -0.57142857 -0.55714286 -0.54285714 -0.52857143 -0.51428571 -0.5 -0.48571429 -0.47142857 -0.45714286 -0.44285714 -0.42857143 -0.41428571 -0.4 -0.38571429 -0.37142857 -0.35714286 -0.34285714 -0.32857143 -0.31428571 -0.3 -0.28571429 -0.27142857 -0.25714286 -0.24285714 -0.22857143 -0.21428571 -0.2 -0.18571429 -0.17142857 -0.15714286 -0.14285714 -0.12857143 -0.11428571 -0.1 -0.08571429 -0.07142857 -0.05714286 -0.04285714 -0.02857143 -0.01428571 0 0 0 0 0 0
  line L11 (5.9179, -7.8951) -> (5.5515, -7.4053)
  arc A23 (5.6309, -6.7225) -> (5.5515, -7.4053) centre (5.9519, -7.1058) ccw
  arc A24 (5.6309, -6.7225) -> (6.0971, -6.3027) centre (0, 0) ccw
  arc A25 (6.7844, -6.2952) -> (6.0971, -6.3027) centre (6.4447, -6.6621) ccw
  line L12 (6.7844, -6.2952) -> (7.2332, -6.7107)
  spline S12 degree 5 poles (7.2332, -6.7107) (7.2376, -6.7148) (7.2465, -6.7228) (7.2602, -6.7343) (7.279, -6.749) (7.3034, -6.7664) (7.3284, -6.7829) (7.3539, -6.799) (7.3795, -6.8149) (7.4053, -6.8306) (7.4313, -6.8461) (7.4575, -6.8614) (7.4839, -6.8763) (7.5106, -6.8909) (7.5376, -6.9051) (7.5649, -6.9189) (7.5925, -6.9325) (7.6202, -6.9457) (7.6481, -6.9588) (7.6762, -6.9716) (7.7044, -6.9843) (7.7328, -6.9967) (7.7614, -7.0088) (7.7901, -7.0207) (7.819, -7.0324) (7.8481, -7.0438) (7.8774, -7.0551) (7.9068, -7.066) (7.9363, -7.0768) (7.966, -7.0874) (7.9958, -7.0978) (8.0258, -7.1079) (8.0559, -7.1179) (8.0862, -7.1276) (8.1165, -7.1372) (8.147, -7.1465) (8.1777, -7.1557) (8.2084, -7.1646) (8.2393, -7.1734) (8.2703, -7.1819) (8.3014, -7.1903) (8.3327, -7.1984) (8.364, -7.2064) (8.3955, -7.2142) (8.427, -7.2218) (8.4587, -7.2292) (8.4905, -7.2364) (8.5224, -7.2435) (8.5544, -7.2503) (8.5865, -7.257) (8.6187, -7.2635) (8.651, -7.2698) (8.6834, -7.2759) (8.7159, -7.2819) (8.7485, -7.2876) (8.7812, -7.2932) (8.814, -7.2986) (8.8469, -7.3038) (8.8798, -7.3089) (8.9129, -7.3137) (8.946, -7.3184) (8.9792, -7.3229) (9.0126, -7.3273) (9.046, -7.3314) (9.0794, -7.3354) (9.113, -7.3392) (9.1466, -7.3429) (9.1804, -7.3464) (9.2141, -7.3496) (9.248, -7.3528) (9.282, -7.3557) (9.3092, -7.3579) (9.3296, -7.3595) (9.3433, -7.3606) (9.3501, -7.3611) knots 0 0 0 0 0 0 0.01428571 0.02857143 0.04285714 0.05714286 0.07142857 0.08571429 0.1 0.11428571 0.12857143 0.14285714 0.15714286 0.17142857 0.18571429 0.2 0.21428571 0.22857143 0.24285714 0.25714286 0.27142857 0.28571429 0.3 0.31428571 0.32857143 0.34285714 0.35714286 0.37142857 0.38571429 0.4 0.41428571 0.42857143 0.44285714 0.45714286 0.47142857 0.48571429 0.5 0.51428571 0.52857143 0.54285714 0.55714286 0.57142857 0.58571429 0.6 0.61428571 0.62857143 0.64285714 0.65714286 0.67142857 0.68571429 0.7 0.71428571 0.72857143 0.74285714 0.75714286 0.77142857 0.78571429 0.8 0.81428571 0.82857143 0.84285714 0.85714286 0.87142857 0.88571429 0.9 0.91428571 0.92857143 0.94285714 0.95714286 0.97142857 0.98571429 1 1 1 1 1 1
  arc A26 (9.3501, -7.3611) -> (9.8901, -6.6178) centre (0, 0) ccw
  spline S13 degree 5 poles (9.8901, -6.6178) (9.8875, -6.6115) (9.8823, -6.5988) (9.8745, -6.5798) (9.864, -6.5546) (9.8507, -6.5233) (9.8373, -6.492) (9.8237, -6.4609) (9.81, -6.4299) (9.7961, -6.399) (9.7821, -6.3683) (9.768, -6.3377) (9.7537, -6.3072) (9.7393, -6.2769) (9.7247, -6.2467) (9.71, -6.2166) (9.6952, -6.1867) (9.6802, -6.1569) (9.665, -6.1272) (9.6498, -6.0977) (9.6344, -6.0683) (9.6188, -6.0391) (9.6031, -6.01) (9.5873, -5.9811) (9.5713, -5.9523) (9.5552, -5.9237) (9.5389, -5.8952) (9.5225, -5.8669) (9.506, -5.8388) (9.4893, -5.8108) (9.4724, -5.7829) (9.4555, -5.7552) (9.4383, -5.7277) (9.4211, -5.7004) (9.4036, -5.6732) (9.3861, -5.6462) (9.3683, -5.6194) (9.3505, -5.5927) (9.3325, -5.5662) (9.3143, -5.5399) (9.296, -5.5138) (9.2775, -5.4878) (9.2589, -5.4621) (9.2402, -5.4365) (9.2212, -5.4112) (9.2022, -5.386) (9.1829, -5.361) (9.1635, -5.3363) (9.144, -5.3117) (9.1243, -5.2873) (9.1044, -5.2632) (9.0844, -5.2393) (9.0642, -5.2156) (9.0438, -5.1922) (9.0232, -5.1691) (9.0025, -5.1461) (8.9816, -5.1234) (8.9606, -5.1009) (8.9394, -5.0786) (8.918, -5.0566) (8.8964, -5.0349) (8.8745, -5.0136) (8.8524, -4.9927) (8.83, -4.9722) (8.8074, -4.952) (8.7846, -4.9321) (8.7617, -4.9124) (8.7387, -4.8929) (8.7156, -4.8737) (8.6921, -4.855) (8.668, -4.8372) (8.6483, -4.8238) (8.633, -4.8144) (8.6227, -4.8084) (8.6175, -4.8055) knots -1 -1 -1 -1 -1 -1 -0.98571429 -0.97142857 -0.95714286 -0.94285714 -0.92857143 -0.91428571 -0.9 -0.88571429 -0.87142857 -0.85714286 -0.84285714 -0.82857143 -0.81428571 -0.8 -0.78571429 -0.77142857 -0.75714286 -0.74285714 -0.72857143 -0.71428571 -0.7 -0.68571429 -0.67142857 -0.65714286 -0.64285714 -0.62857143 -0.61428571 -0.6 -0.58571429 -0.57142857 -0.55714286 -0.54285714 -0.52857143 -0.51428571 -0.5 -0.48571429 -0.47142857 -0.45714286 -0.44285714 -0.42857143 -0.41428571 -0.4 -0.38571429 -0.37142857 -0.35714286 -0.34285714 -0.32857143 -0.31428571 -0.3 -0.28571429 -0.27142857 -0.25714286 -0.24285714 -0.22857143 -0.21428571 -0.2 -0.18571429 -0.17142857 -0.15714286 -0.14285714 -0.12857143 -0.11428571 -0.1 -0.08571429 -0.07142857 -0.05714286 -0.04285714 -0.02857143 -0.01428571 0 0 0 0 0 0
  line L13 (8.6175, -4.8055) -> (8.0836, -4.507)
  arc A27 (7.8784, -3.851) -> (8.0836, -4.507) centre (8.3276, -4.0706) ccw
  arc A28 (7.8784, -3.851) -> (8.1335, -3.2779) centre (0, 0) ccw
  arc A29 (8.7583, -2.9915) -> (8.1335, -3.2779) centre (8.5973, -3.4648) ccw
  line L14 (8.7583, -2.9915) -> (9.3374, -3.1885)
  spline S14 degree 5 poles (9.3374, -3.1885) (9.343, -3.1904) (9.3544, -3.1941) (9.3716, -3.1992) (9.3948, -3.2049) (9.4241, -3.2108) (9.4537, -3.2158) (9.4835, -3.2202) (9.5134, -3.2242) (9.5433, -3.228) (9.5734, -3.2316) (9.6035, -3.2349) (9.6337, -3.2378) (9.6641, -3.2403) (9.6945, -3.2423) (9.7251, -3.2438) (9.7558, -3.245) (9.7865, -3.2458) (9.8173, -3.2464) (9.8482, -3.2467) (9.8791, -3.2468) (9.9101, -3.2466) (9.9411, -3.246) (9.9722, -3.2452) (10.0034, -3.2441) (10.0346, -3.2428) (10.0659, -3.2411) (10.0972, -3.2392) (10.1286, -3.237) (10.16, -3.2346) (10.1915, -3.2319) (10.223, -3.229) (10.2545, -3.2259) (10.2861, -3.2225) (10.3178, -3.2189) (10.3494, -3.215) (10.3811, -3.2109) (10.4129, -3.2065) (10.4446, -3.202) (10.4764, -3.1972) (10.5083, -3.1921) (10.5401, -3.1869) (10.572, -3.1814) (10.6039, -3.1758) (10.6359, -3.1699) (10.6678, -3.1637) (10.6998, -3.1574) (10.7318, -3.1509) (10.7638, -3.1441) (10.7959, -3.1372) (10.8279, -3.13) (10.86, -3.1226) (10.8921, -3.115) (10.9242, -3.1072) (10.9563, -3.0992) (10.9884, -3.091) (11.0206, -3.0826) (11.0527, -3.074) (11.0849, -3.0652) (11.1171, -3.0562) (11.1493, -3.047) (11.1815, -3.0376) (11.2137, -3.0281) (11.2459, -3.0183) (11.2781, -3.0083) (11.3103, -2.9981) (11.3425, -2.9878) (11.3747, -2.9772) (11.4069, -2.9665) (11.4391, -2.9556) (11.4713, -2.9445) (11.4971, -2.9354) (11.5164, -2.9286) (11.5293, -2.9239) (11.5358, -2.9216) knots 0 0 0 0 0 0 0.01428571 0.02857143 0.04285714 0.05714286 0.07142857 0.08571429 0.1 0.11428571 0.12857143 0.14285714 0.15714286 0.17142857 0.18571429 0.2 0.21428571 0.22857143 0.24285714 0.25714286 0.27142857 0.28571429 0.3 0.31428571 0.32857143 0.34285714 0.35714286 0.37142857 0.38571429 0.4 0.41428571 0.42857143 0.44285714 0.45714286 0.47142857 0.48571429 0.5 0.51428571 0.52857143 0.54285714 0.55714286 0.57142857 0.58571429 0.6 0.61428571 0.62857143 0.64285714 0.65714286 0.67142857 0.68571429 0.7 0.71428571 0.72857143 0.74285714 0.75714286 0.77142857 0.78571429 0.8 0.81428571 0.82857143 0.84285714 0.85714286 0.87142857 0.88571429 0.9 0.91428571 0.92857143 0.94285714 0.95714286 0.97142857 0.98571429 1 1 1 1 1 1
  arc A30 (11.5358, -2.9216) -> (11.7268, -2.023) centre (0, 0) ccw